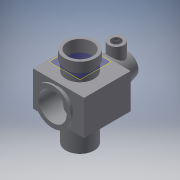
# Autodesk Inventor part: Carburetor Housing
Saved by Autodesk Inventor 2016 (Build 200138000, 138)
## iProperties
Created: 2012-08-08
Part Number: Carburetor Housing
Material: Generic
Document SubType Name: Modeling
Designer: John
Density: 1 g/cm^3
Appearance: Default
Author: John
Autodesk Inventor part; units mm, degrees
note: some values were not read from the file. Chosen so that the rebuilt part matches the saved one: direction of "Hole2"; direction of "Hole4".
ref_plane "YZ Plane" through (0, 0, 0) normal (1, 0, 0) x (0, 1, 0)
ref_plane "XZ Plane" through (0, 0, 0) normal (0, 1, 0) x (-1, 0, 0)
ref_plane "XY Plane" through (0, 0, 0) normal (0, 0, 1) x (1, 0, 0)
sketch "Sketch1" plane through (0, 0, 0) normal (0, 0, 1) x (1, 0, 0)
  line L0 (0, 0) -> (53.975, 0)
  line L1 (53.975, 0) -> (53.975, 49.276)
  line L2 (53.975, 49.276) -> (0, 49.276)
  line L3 (0, 49.276) -> (0, 0)
  dimension "d0" = 53.975
  dimension "d1" = 49.276
  constraints: 8 end point, 2 parallel, 1 horizontal, 1 perpendicular
  measures "d0" distance of L2.end L1.end
  measures "d1" distance of L1.end L0.end
extrude "Extrusion1" add sketch "Sketch1" along normal blind 36.9062
sketch "Sketch2" plane through (0, 0, 0) normal (0, 0, -1) x (-1, 0, 0)
  line L0 (0, 0) -> (-53.975, 0) projected
  line L1 (-53.975, 49.276) -> (0, 49.276) projected
  line L2 (-26.9875, 0) -> (-26.9875, 49.276) construction
  circle A0 centre (-26.9875, 22.733) radius 14.9352
  dimension "d4" = 29.8704
  dimension "d14" = 22.733
  constraints: 2 end point, 2 midpoint, 1 centre point, 1 point on line
  measures "d4" diameter of A0
  measures "d14" distance from line of L0 A0.centre
extrude "Extrusion2" add sketch "Sketch2" along normal blind 28.7528
sketch "Sketch3" plane through (0, 0, 0) normal (0, -1, 0) x (1, 0, 0)
  line L0 (0, 0) -> (53.975, 36.9062) construction
  circle A0 centre (26.9875, 18.4531) radius 15.24
  dimension "d8" = 30.48
  constraints: 2 end point, 2 midpoint, 1 centre point
  measures "d8" diameter of A0
extrude "Extrusion3" add sketch "Sketch3" along normal blind 6.35
sketch "Sketch4" plane through (26.9875, -6.35, 18.4531) normal (0, -1, 0) x (1, 0, 0)
  circle A0 centre (0, 0) radius 15.24 projected
  circle A1 centre (0, 0) radius 19.5072
  point P0 (-26.9875, -18.4531)
  dimension "d11" = 39.0144
  constraints: 1 centre point, 1 coincident
  measures "d11" diameter of A1
extrude "Extrusion4" add sketch "Sketch4" against normal blind 1.905 contours A0 | A1
sketch "Sketch5" plane through (0, 0, 36.9062) normal (0, 0, 1) x (1, 0, 0)
  circle A0 centre (26.9875, 22.733) radius 14.9352 projected
  circle A1 centre (26.9875, 22.733) radius 21.9462
  constraints: 1 centre point, 1 coincident
extrude "Extrusion5" add sketch "Sketch5" along normal blind 10.6934 contours A0
sketch "Sketch7" plane through (26.9875, 22.733, 47.5996) normal (0, 0, 1) x (1, 0, 0)
  circle A0 centre (0, 0) radius 14.9352 projected
  circle A1 centre (0, 0) radius 16.4592
  point P0 (-26.9875, -22.733)
  dimension "d18" = 32.9184
  constraints: 1 centre point, 1 coincident
  measures "d18" diameter of A1
extrude "Extrusion6" add sketch "Sketch7" along normal blind 9.144 contours A0 | A1
sketch "Sketch8" plane through (0, 49.276, 0) normal (0, 1, 0) x (1, 0, 0)
  line L0 (53.975, 0) -> (0, 0) projected
  line L1 (53.975, 0) -> (0, -36.9062) construction
  circle A0 centre (26.9875, -18.4531) radius 17.9451
  dimension "d21" = 0.508
  constraints: 2 end point, 1 centre point, 1 midpoint
  measures "d21" distance edge to line of A0 L0
extrude "Extrusion7" add sketch "Sketch8" along normal blind 23.622 draft -15
ref_plane "Work Plane1" through (26.9875, 22.733, 45.1612) normal (0, 0, -1) x (-1, 0, 0)
sketch "Sketch9" plane through (26.9875, 22.733, 45.1612) normal (0, 0, -1) x (-1, 0, 0)
  line L0 (0, -29.083) -> (0, 38.354)
  circle A0 centre (0, 38.354) radius 7.9375
  line L1 (19.5072, -29.083) -> (-19.5072, -29.083) projected
  dimension "d25" = 67.437
  dimension "d26" = 15.875
  constraints: 2 end point, 1 centre point, 1 coincident, 1 midpoint, 1 vertical
  measures "d25" distance of L0.start L0.end
  measures "d26" diameter of A0
extrude "Extrusion8" add sketch "Sketch9" along normal up to next
sketch "Sketch10" plane through (26.9875, -6.35, 18.4531) normal (0, -1, 0) x (1, 0, 0)
  circle A0 centre (0, 0) radius 19.5072 projected
  point P0 (-26.9875, -18.4531)
hole "Hole1" at (26.9875, -6.35, 18.4531) direction (0, 1, 0) diameter 29.718 depth 47.244
sketch "Sketch11" plane through (26.9875, 22.733, -28.7528) normal (0, 0, -1) x (-1, 0, 0)
  circle A0 centre (0, 0) radius 14.9352 projected
  point P0 (26.9875, -22.733)
hole "Hole2" at (26.9875, 22.733, -28.7528) direction (0, 0, 1) diameter 25.4 end up to surface
sketch "Sketch12" plane through (26.9875, 22.733, 56.7436) normal (0, 0, 1) x (1, 0, 0)
  circle A0 centre (0, 0) radius 16.4592 projected
  circle A1 centre (0, 0) radius 13.1826
  point P0 (-26.9875, -22.733)
  dimension "d43" = 26.3652
  constraints: 1 centre point, 1 coincident
  measures "d43" diameter of A1
extrude "Extrusion9" cut sketch "Sketch12" against normal up to surface draft -5 contours A1
sketch "Sketch13" plane through (26.9875, 72.898, 18.4531) normal (0, 1, 0) x (1, 0, 0)
  circle A0 centre (0, 0) radius 11.6156 projected
  point P0 (-26.9875, 18.4531)
hole "Hole3" at (26.9875, 72.898, 18.4531) direction (0, -1, 0) diameter 19.05 end through all
sketch "Sketch14" plane through (26.9875, 61.087, 45.1612) normal (0, 0, 1) x (1, 0, 0)
  circle A0 centre (0, 0) radius 7.9375 projected
  point P0 (-26.9875, -61.087)
hole "Hole4" at (26.9875, 61.087, 45.1612) direction (0, 0, -1) diameter 9.7282 end up to surface thread size "7/16-20 UNF" class "2B" standard "ANSI Unified Screw Threads"
body "Solid1"
